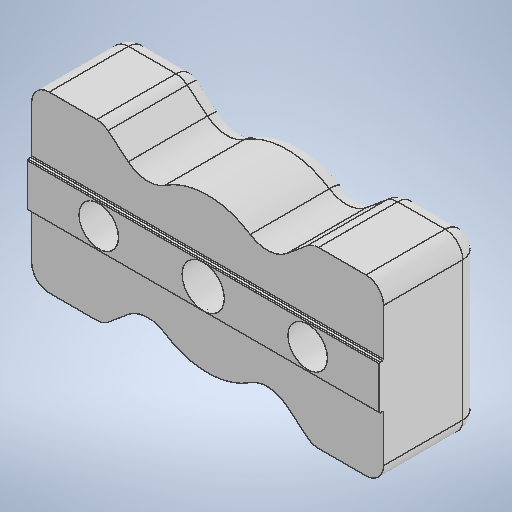
# Autodesk Inventor part: Base_Mount_Pedals
Saved by Autodesk Inventor 2026.2 (Build 302298000, 298)
## iProperties
Created: 2026-03-23
Part Number: Base_Mount_Pedals
Material: Generic
Document SubType Name: Modeling
Designer: Paco Ariel
Density: 1 g/cm^3
Appearance: Default
Author: Paco Ariel
Autodesk Inventor part; units mm, degrees
ref_plane "YZ Plane" through (0, 0, 0) normal (1, 0, 0) x (0, 1, 0)
ref_plane "XZ Plane" through (0, 0, 0) normal (0, 1, 0) x (-1, 0, 0)
ref_plane "XY Plane" through (0, 0, 0) normal (0, 0, 1) x (1, 0, 0)
sketch "Sketch1" plane through (0, 0, 0) normal (0, 0, 1) x (1, 0, 0)
  line L0 (-40, 19.775) -> (40, 19.775)
  line L1 (40, 19.775) -> (40, -19.775)
  line L2 (40, -19.775) -> (-40, -19.775)
  line L3 (-40, -19.775) -> (-40, 19.775)
  line L4 (-40, 19.775) -> (40, -19.775) construction
  line L5 (40, 19.775) -> (-40, -19.775) construction
  line L6 (40, -5) -> (-40, -5)
  line L7 (-40, -5) -> (-40, 5)
  line L8 (-40, 5) -> (40, 5)
  line L9 (40, 5) -> (40, -5)
  line L10 (40, -5) -> (-40, 5) construction
  line L11 (-40, -5) -> (40, 5) construction
  line L12 (23.75, 0) -> (-23.75, 0)
  circle A0 centre (-23.75, 0) radius 4.5
  circle A1 centre (23.75, 0) radius 4.5
  circle A2 centre (0, 0) radius 8
  point P0 (40, 5)
  point P1 (-40, -5)
  point P2 (40, -5)
  point P3 (-6.245, -5)
  point P4 (6.245, -5)
  point P5 (6.245, 5)
  point P6 (-6.245, 5)
  dimension "d0" = 80
  dimension "d1" = 39.55
  dimension "d3" = 10
  dimension "d9" = 80
  dimension "d10" = 47.5
  dimension "d11" = 9
  dimension "d12" = 9
  dimension "d15" = 16
  dimension "d42" = 19.775
  dimension "d43" = 0
  constraints: 26 end point, 5 midpoint, 4 parallel, 3 centre point, 3 coincident, 3 horizontal, 2 perpendicular
  measures "d0" distance of L1.end L2.end
  measures "d1" distance of L0.end L1.end
  measures "d3" distance of L6.end L7.end
  measures "d9" distance between parallel lines of L9 L7
  measures "d10" distance of L12.start L12.end
  measures "d11" diameter of A0
  measures "d12" diameter of A1
  measures "d15" diameter of A2
  measures "d42" distance between parallel lines of L0 L12
  measures "d43" distance between parallel lines of L3 L7
extrude "Extrusion1" add sketch "Sketch1" along normal blind 1 contours L8 A2 L6 L3 | L1 L6 A2 L8 | L8 A2 L12 | A2 L12 L6
extrude "Extrusion2" add sketch "Sketch1" against normal blind 6
fillet "Fillet1" radius 0.2 4 edges at (0, 5, 0) (0, 5, 1) (0, -5, 1) (0, -5, 0)
sketch "Sketch2" plane through (0, 0, -6) normal (0, 0, -1) x (-1, 0, 0)
  circle A0 centre (23.75, 0) radius 4.5 projected
  circle A1 centre (-23.75, 0) radius 4.5 projected
  circle A2 centre (23.75, 0) radius 7
  circle A3 centre (-23.75, 0) radius 7
  line L0 (-40, -19.775) -> (40, -19.775) projected
  line L1 (-40, 19.775) -> (-40, -19.775) projected
  line L2 (40, 19.775) -> (-40, 19.775) projected
  line L3 (40, -19.775) -> (40, 19.775) projected
  point P0 (0, 0)
  dimension "d16" = 14
  dimension "d17" = 14
  constraints: 2 centre point, 2 coincident
  measures "d16" diameter of A2
  measures "d17" diameter of A3
extrude "Extrusion3" add sketch "Sketch2" along normal blind 16 contours L1 L2 L3 L0
sketch "Sketch3" plane through (0, 0, -22) normal (0, 0, -1) x (-1, 0, 0)
  circle A0 centre (0, 0) radius 5.15
  dimension "d21" = 10.3
  constraints: 1 centre point, 1 coincident
  measures "d21" diameter of A0
extrude "Extrusion4" cut sketch "Sketch3" against normal blind 10
sketch "Sketch4" plane through (0, 0, -22) normal (0, 0, -1) x (-1, 0, 0)
  circle A0 centre (0, 0) radius 5.15 projected
  circle A1 centre (0, 0) radius 7.25
  dimension "d24" = 14.5
  constraints: 1 centre point, 1 coincident
  measures "d24" diameter of A1
extrude "Extrusion5" add sketch "Sketch4" along normal blind 1
chamfer "Chamfer1" distance 1 distance2 1 1 edges at (7.25, 0, -22) measured on face at (-0.2913, -15.5824, -22)
sketch "Sketch5" plane through (0, 0, -12) normal (0, 0, -1) x (-1, 0, 0)
  circle A0 centre (0, 0) radius 4.8
  dimension "d30" = 9.6
  constraints: 1 centre point, 1 coincident
  measures "d30" diameter of A0
extrude "Extrusion6" cut sketch "Sketch5" against normal blind 20
sketch "Sketch6" plane through (0, 0, -22) normal (0, 0, -1) x (-1, 0, 0)
  circle A0 centre (0, 0) radius 17.5
  circle A1 centre (23.75, 0) radius 7 projected
  circle A2 centre (-23.75, 0) radius 7 projected
  line L0 (40, -19.775) -> (40, 19.775) projected
  line L1 (40, 19.775) -> (-40, 19.775) projected
  line L2 (-40, 19.775) -> (-40, -19.775) projected
  line L3 (-40, -19.775) -> (40, -19.775) projected
  circle A3 centre (0, 0) radius 8.25 projected
  line L4 (-23.75, 0) -> (-23.75, 19.775)
  line L5 (13.4485, 11.1977) -> (23.75, 19.775)
  line L6 (-40, 19.775) -> (40, 19.775) projected
  line L7 (-23.75, 19.775) -> (-13.4485, 11.1977)
  dimension "d33" = 35
  constraints: 6 end point, 2 point on circle, 2 point on line, 1 centre point, 1 coincident, 1 vertical
  measures "d33" diameter of A0
extrude "Extrusion7" cut sketch "Sketch6" against normal through all contours A0 L7 L1 L5
mirror "Mirror1" about plane through (0, 0, 0) normal (0, 1, 0) of "Extrusion7"
fillet "Fillet3" radius 7 4 edges at (13.4485, 11.1977, -11) (-13.4485, 11.1977, -11) (13.4485, -11.1977, -11) (-13.4485, -11.1977, -11)
fillet "Fillet4" radius 4 8 edges at (23.75, -19.775, -11) (40, -19.775, -11) (40, 19.775, -11) (23.75, 19.775, -11) (-23.75, 19.775, -11) (-40, 19.775, -11) (-40, -19.775, -11) (-23.75, -19.775, -11)
fillet "Fillet5" radius 4 24 edges at (38.8284, 18.6034, -22) (40, 0, -22) (38.8284, -18.6034, -22) (30.5986, -19.775, -22) (23.8363, -19.5364, -22) (20.3404, -16.9361, -22) (13.9404, -13.4128, -22) (0, -17.5, -22) (-13.9404, -13.4128, -22) (-20.3404, -16.9361, -22) (-23.8363, -19.5364, -22) (-30.5986, -19.775, -22) (-38.8284, -18.6034, -22) (-40, 0, -22) (-38.8284, 18.6034, -22) (-30.5986, 19.775, -22) (-23.8363, 19.5364, -22) (-20.3404, 16.9361, -22) (-13.9404, 13.4128, -22) (0, 17.5, -22) (13.9404, 13.4128, -22) (20.3404, 16.9361, -22) (23.8363, 19.5364, -22) (30.5986, 19.775, -22)
chamfer "Chamfer2" distance 0.5 angle 45 2 edges at (-16.75, 0, -22) (30.75, 0, -22)
equation "\"d9\" = d0"
body "Solid1"
